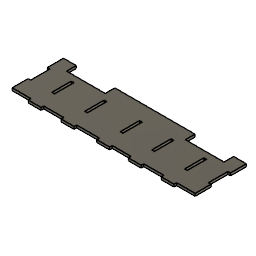
Muur Lang (Autodesk Fusion 360 design; units mm, degrees)
part number: 2026-03-19-13-11-23-386
Autodesk Fusion 360 part; units mm, degrees
sketch "Sketch1" plane through (0, 0, 0) normal (0, 0, 1) x (1, 0, 0)
  line L0 (3.7286, -31.8797) -> (3.7286, -35.8797)
  line L1 (3.7286, -35.8797) -> (-16.2714, -35.8797)
  line L2 (-16.2714, -35.8797) -> (-16.2714, -31.8797)
  line L3 (54.8886, -31.8797) -> (54.8886, -35.8797)
  line L4 (54.8886, -35.8797) -> (34.8886, -35.8797)
  line L5 (34.8886, -35.8797) -> (34.8886, -31.8797)
  line L6 (110.3886, -31.8797) -> (110.3886, -35.8797)
  line L7 (110.3886, -35.8797) -> (90.3886, -35.8797)
  line L8 (90.3886, -35.8797) -> (90.3886, -31.8797)
  line L9 (159.5486, -31.8797) -> (159.5486, -35.8797)
  line L10 (159.5486, -35.8797) -> (139.5486, -35.8797)
  line L11 (139.5486, -35.8797) -> (139.5486, -31.8797)
  line L12 (190.7086, -31.8797) -> (190.7086, -35.8797)
  line L13 (190.7086, -35.8797) -> (210.7086, -35.8797)
  line L14 (210.7086, -35.8797) -> (210.7086, -31.8797)
  line L15 (239.5686, -31.8797) -> (235.3824, -31.8797)
  line L16 (235.3824, -31.8797) -> (210.7086, -31.8797)
  line L17 (190.7086, -31.8797) -> (187.1012, -31.8797)
  line L18 (187.1012, -31.8797) -> (159.5486, -31.8797)
  line L19 (139.5486, -31.8797) -> (110.3886, -31.8797)
  line L20 (90.3886, -31.8797) -> (54.8886, -31.8797)
  line L21 (34.8886, -31.8797) -> (29.9892, -31.8797)
  line L22 (29.9892, -31.8797) -> (3.7286, -31.8797)
  line L23 (-16.2714, -31.8797) -> (-45.4314, -31.8797)
  line L24 (159.5686, 48.1203) -> (159.5686, 33.1203)
  line L25 (159.5686, 33.1203) -> (219.5686, 33.1203)
  line L26 (219.5686, 33.1203) -> (219.5686, 48.1203)
  line L27 (34.5686, 48.1203) -> (34.5686, 33.1203)
  line L28 (34.5686, 33.1203) -> (-25.4314, 33.1203)
  line L29 (-25.4314, 33.1203) -> (-25.4314, 48.1203)
  line L30 (239.5686, 48.1203) -> (219.5686, 48.1203)
  line L31 (159.5686, 48.1203) -> (34.5686, 48.1203)
  line L32 (-25.4314, 48.1203) -> (-45.4314, 48.1203)
  line L33 (-45.4314, -6.8797) -> (-41.4314, -6.8797)
  line L34 (-41.4314, -6.8797) -> (-41.4314, 23.1203)
  line L35 (-41.4314, 23.1203) -> (-45.4314, 23.1203)
  line L36 (-45.4314, -31.8797) -> (-45.4314, -27.5346)
  line L37 (-45.4314, -27.5346) -> (-45.4314, -6.8797)
  line L38 (-45.4314, 23.1203) -> (-45.4314, 26.6822)
  line L39 (-45.4314, 26.6822) -> (-45.4314, 48.1203)
  line L40 (-45.4314, -6.8797) -> (-41.4314, -6.8797)
  line L41 (-41.4314, -6.8797) -> (-41.4314, 23.1203)
  line L42 (-45.4314, 23.1203) -> (-45.4314, 26.6822)
  line L43 (-41.4314, 23.1203) -> (-45.4314, 23.1203)
  line L44 (239.5686, 23.1203) -> (235.5686, 23.1203)
  line L45 (235.5686, -6.8797) -> (239.5686, -6.8797)
  line L46 (239.5686, 23.1203) -> (235.5686, 23.1203)
  line L47 (235.5686, -6.8797) -> (239.5686, -6.8797)
  line L48 (235.5686, 23.1203) -> (235.5686, -6.8797)
  line L49 (239.5686, 23.1203) -> (239.5686, 48.1203)
  line L50 (239.5686, -31.8797) -> (239.5686, -30.1367)
  line L51 (239.5686, -30.1367) -> (239.5686, -6.8797)
  line L52 (-8.2714, -6.8797) -> (-4.2714, -6.8797)
  line L53 (-4.2714, -6.8797) -> (-4.2714, 23.1203)
  line L54 (-4.2714, 23.1203) -> (-8.2714, 23.1203)
  line L55 (-8.2714, 23.1203) -> (-8.2714, -6.8797)
  line L56 (42.8886, -6.8797) -> (46.8886, -6.8797)
  line L57 (46.8886, -6.8797) -> (46.8886, 23.1203)
  line L58 (46.8886, 23.1203) -> (42.8886, 23.1203)
  line L59 (42.8886, 23.1203) -> (42.8886, -6.8797)
  line L60 (98.0886, -6.8797) -> (102.0886, -6.8797)
  line L61 (102.0886, -6.8797) -> (102.0886, 23.1203)
  line L62 (102.0886, 23.1203) -> (98.0886, 23.1203)
  line L63 (98.0886, 23.1203) -> (98.0886, -6.8797)
  line L64 (147.2486, -6.8797) -> (151.2486, -6.8797)
  line L65 (151.2486, -6.8797) -> (151.2486, 23.1203)
  line L66 (151.2486, 23.1203) -> (147.2486, 23.1203)
  line L67 (147.2486, 23.1203) -> (147.2486, -6.8797)
  line L68 (198.4086, -6.8797) -> (202.4086, -6.8797)
  line L69 (202.4086, -6.8797) -> (202.4086, 23.1203)
  line L70 (202.4086, 23.1203) -> (198.4086, 23.1203)
  line L71 (198.4086, 23.1203) -> (198.4086, -6.8797)
  constraint vertical L0
  constraint vertical L2
  constraint vertical L3
  constraint vertical L5
  constraint vertical L6
  constraint vertical L8
  constraint vertical L9
  constraint vertical L11
  constraint vertical L12
  constraint vertical L14
  constraint perpendicular L14 L16
  constraint perpendicular L9 L18
  constraint perpendicular L6 L19
  constraint perpendicular L3 L20
  constraint perpendicular L0 L22
  constraint vertical L24
  constraint horizontal L25
  constraint vertical L26
  constraint vertical L27
  constraint horizontal L28
  constraint vertical L29
  constraint perpendicular L26 L30
  constraint perpendicular L27 L31
  constraint horizontal L33
  constraint vertical L34
  constraint horizontal L35
  constraint perpendicular L23 L36
  constraint perpendicular L33 L37
  constraint perpendicular L32 L39
  constraint horizontal L40
  constraint vertical L41
  constraint horizontal L43
  constraint horizontal L47
  constraint horizontal L44
  constraint horizontal L45
  constraint horizontal L46
  constraint perpendicular L45 L48
  constraint perpendicular L30 L49
  constraint perpendicular L15 L50
  constraint perpendicular L47 L51
  constraint horizontal L52
  constraint vertical L53
  constraint horizontal L54
  constraint vertical L55
  constraint horizontal L56
  constraint vertical L57
  constraint horizontal L58
  constraint vertical L59
  constraint horizontal L60
  constraint vertical L61
  constraint horizontal L62
  constraint vertical L63
  constraint horizontal L64
  constraint vertical L65
  constraint horizontal L66
  constraint vertical L67
  constraint horizontal L68
  constraint vertical L69
  constraint horizontal L70
  constraint vertical L71
extrude "Extrude1" add sketch "Sketch1" along normal blind 4
